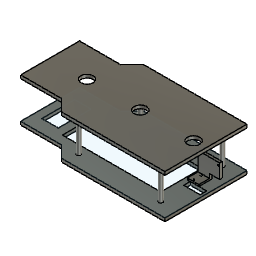
secondbody_final (Autodesk Fusion 360 design; units mm, degrees)
Autodesk Fusion 360 part; units mm, degrees
sketch "Sketch1" plane through (0, 0, 0) normal (0, 0, 1) x (1, 0, 0)
  line L0 (70, 50) -> (-70, 50)
  line L1 (-70, 50) -> (-70, -50)
  line L2 (-70, -50) -> (70, -50)
  line L3 (70, -50) -> (70, 50)
  line L4 (70, 50) -> (-70, -50) construction
  line L5 (-70, 50) -> (70, -50) construction
  line L6 (-70, 35.8825) -> (-120, 35.8825)
  line L7 (-120, 35.8825) -> (-120, -35.8857)
  line L8 (-120, -35.8857) -> (-70, -35.8857)
  line L9 (-70, -35.8857) -> (-70, 35.8825)
  line L10 (-70, 35.8825) -> (-120, -35.8857) construction
  line L11 (-120, 35.8825) -> (-70, -35.8857) construction
  point P0 (-95, -0.0016)
  dimension "d1" = 140
  dimension "d44" = 100
  dimension "d45" = 50
  constraint horizontal L0
  constraint perpendicular L0 L1
  constraint parallel L0 L2
  constraint parallel L1 L3
  constraint coincident L4 origin
  constraint coincident L5 origin
  constraint horizontal L6
  constraint perpendicular L6 L7
  constraint parallel L6 L8
  constraint parallel L7 L9
  constraint coincident L10 P0
  constraint coincident L11 P0
  constraint coincident L1 L6.start
  measures "d1" distance of L1.end L2.end
  measures "d44" distance of L0.start L2.end
  measures "d45" distance of L7.end L8.end
extrude "Extrude1" add sketch "Sketch1" along normal blind 4 makes body 1
sketch "Sketch3" plane through (0, 0, 4) normal (0, 0, 1) x (-1, 0, 0)
  line L0 (70, -50) -> (70, -35.8825)
  line L1 (70, 35.8857) -> (70, 50)
  line L2 (70, 50) -> (-70, 50)
  line L3 (-70, 50) -> (-70, -50)
  line L4 (-70, -50) -> (70, -50)
  line L5 (70, -35.8825) -> (120, -35.8825)
  line L6 (120, -35.8825) -> (120, 35.8857)
  line L7 (120, 35.8857) -> (70, 35.8857)
  line L8 (-40, -25) -> (80, -25)
  line L9 (80, -25) -> (80, 25)
  line L10 (80, 25) -> (-40, 25)
  line L11 (-40, 25) -> (-40, -25)
  line L12 (-40, -25) -> (80, 25) construction
  line L13 (80, -25) -> (-40, 25) construction
  point P0 (20, 0)
  dimension "d54" = 120
  dimension "d55" = 50
  constraint horizontal L8
  constraint perpendicular L8 L9
  constraint parallel L8 L10
  constraint parallel L9 L11
  constraint coincident L12 P0
  constraint coincident L13 P0
  measures "d54" distance of L9.end L10.end
  measures "d55" distance of L8.end L9.end
sketch "Sketch8" plane through (0, 0, 4) normal (0, 0, 1) x (-1, 0, 0)
  line L0 (-70, 50) -> (-70, -50)
  line L1 (-70, -50) -> (70, -50)
  line L2 (70, -50) -> (70, -35.8825)
  line L3 (70, -35.8825) -> (120, -35.8825)
  line L4 (120, -35.8825) -> (120, 35.8857)
  line L5 (120, 35.8857) -> (70, 35.8857)
  line L6 (70, 35.8857) -> (70, 50)
  line L7 (70, 50) -> (-70, 50)
  line L8 (90, 20) -> (90, -20)
  line L9 (90, -20) -> (110, -20)
  line L10 (110, -20) -> (110, 20)
  line L11 (110, 20) -> (90, 20)
  line L12 (90, 20) -> (110, -20) construction
  line L13 (90, -20) -> (110, 20) construction
  point P0 (100, 0)
  dimension "d46" = 40
  dimension "d47" = 20
  constraint perpendicular L8 L9
  constraint parallel L8 L10
  constraint parallel L9 L11
  constraint coincident L12 P0
  constraint coincident L13 P0
  measures "d46" distance of L9.end L10.end
  measures "d47" distance of L8.end L9.end
extrude "Extrude9" cut sketch "Sketch8" against normal blind 45 contours L8 L9 L10 L11 bodies 1
chamfer "Chamfer5" distance 14.1 angle 45 1 edges at (-70, -50, 2) on bodies 1
chamfer "Chamfer6" distance 14.1 angle 45 1 edges at (-70, 50, 2) on bodies 1
sketch "Sketch9" plane through (0, 0, 4) normal (0, 0, 1) x (-1, 0, 0)
  line L0 (55.9, -50) -> (70, -35.9)
  line L1 (70, -35.9) -> (70, -35.8825)
  line L2 (70, -35.8825) -> (120, -35.8825)
  line L3 (120, -35.8825) -> (120, 35.8857)
  line L4 (120, 35.8857) -> (70, 35.8857)
  line L5 (70, 35.8857) -> (70, 35.9)
  line L6 (70, 35.9) -> (55.9, 50)
  line L7 (55.9, 50) -> (-70, 50)
  line L8 (-70, 50) -> (-70, -50)
  line L9 (-70, -50) -> (55.9, -50)
  line L10 (90, -20) -> (90, 20)
  line L11 (90, 20) -> (110, 20)
  line L12 (110, 20) -> (110, -20)
  line L13 (110, -20) -> (90, -20)
extrude "Extrude10" cut sketch "Sketch3" against normal blind 70 contours L8 L9 L10 L11 bodies 1
sketch "Sketch10" plane through (0, 0, 4) normal (0, 0, 1) x (-1, 0, 0)
  line L0 (-44.5, 0) -> (-54.5, 0)
  line L1 (-54.5, 0) -> (-54.5, -20)
  line L2 (-54.5, -20) -> (-44.5, -20)
  line L3 (-44.5, -20) -> (-44.5, 0)
  line L4 (-44.5, 0) -> (-54.5, -20) construction
  line L5 (-54.5, 0) -> (-44.5, -20) construction
  point P0 (-49.5, -10)
  dimension "d58" = 10
  dimension "d59" = 20
  constraint horizontal L0
  constraint perpendicular L0 L1
  constraint parallel L0 L2
  constraint parallel L1 L3
  constraint coincident L4 P0
  constraint coincident L5 P0
  measures "d58" distance of L1.end L2.end
  measures "d59" distance of L0.end L1.end
extrude "Extrude1'" add sketch "Sketch10" along normal blind 2 separate body makes body 2 in component "Component"
sketch "Sketch11" plane through (0, 0, 4) normal (0, 0, 1) x (-1, 0, 0)
  line L0 (-47, 4) -> (-67, 4)
  line L1 (-67, 4) -> (-67, -4)
  line L2 (-67, -4) -> (-47, -4)
  line L3 (-47, -4) -> (-47, 4)
  line L4 (-47, 4) -> (-67, -4) construction
  line L5 (-67, 4) -> (-47, -4) construction
  point P0 (-57, 0)
  dimension "d62" = 20
  dimension "d63" = 8
  constraint horizontal L0
  constraint perpendicular L0 L1
  constraint parallel L0 L2
  constraint parallel L1 L3
  constraint coincident L4 P0
  constraint coincident L5 P0
  measures "d62" distance of L1.end L2.end
  measures "d63" distance of L0.end L1.end
extrude "Extrude11" cut sketch "Sketch11" against normal blind 14 bodies 1
sketch "Sketch12" plane through (0, 0, 6) normal (0, 0, 1) x (-1, 0, 0)
  line L0 (-44.5, -20) -> (-44.5, 0)
  line L1 (-44.5, 0) -> (-54.5, 0)
  line L2 (-54.5, 0) -> (-54.5, -20)
  line L3 (-54.5, -20) -> (-44.5, -20)
  circle A0 centre (-49.5, -6) radius 1
  circle A1 centre (-49.5, -15) radius 1
  dimension "d66" = 2
  dimension "d67" = 2
  measures "d66" diameter of A0
  measures "d67" diameter of A1
extrude "Extrude12" [suppressed]
extrude "Extrude2" cut sketch "Sketch12" against normal blind 2 contours A0 | A1 bodies 2 in component "Component"
sketch "Sketch13" plane through (0, 0, 6) normal (0, 0, 1) x (-1, 0, 0)
  circle A0 centre (-49.5, -15) radius 1
  circle A1 centre (-49.5, -6) radius 1
  line L0 (-44.5, -20) -> (-44.5, 0)
  line L1 (-44.5, 0) -> (-54.5, 0)
  line L2 (-54.5, 0) -> (-54.5, -20)
  line L3 (-54.5, -20) -> (-44.5, -20)
  line L4 (-54.5, -20) -> (-44.5, -20)
  line L5 (-44.5, -20) -> (-44.5, -16.9663)
  line L6 (-44.5, -16.9663) -> (-54.5, -16.9663)
  line L7 (-54.5, -16.9663) -> (-54.5, -20)
  constraint horizontal L4
  constraint vertical L5
  constraint horizontal L6
  constraint vertical L7
  constraint coincident L0 L5.end
  constraint coincident L2.end L3.start
extrude "Extrude3" add sketch "Sketch13" along normal blind 35 contours L0 L2 L3 L4 L5 L6 L7 bodies 2 in component "Component"
sketch "Sketch14" plane through (54.5, 0, 0) normal (1, 0, 0) x (0, 1, 0)
  line L0 (0, 4) -> (20, 4)
  line L1 (20, 4) -> (20, 41)
  line L2 (20, 41) -> (16.9663, 41)
  line L3 (16.9663, 41) -> (16.9663, 6)
  line L4 (16.9663, 6) -> (0, 6)
  line L5 (0, 6) -> (0, 4)
  line L6 (16.9663, 41) -> (20, 41)
  line L7 (20, 41) -> (20, 11)
  line L8 (20, 11) -> (16.9663, 11)
  line L9 (16.9663, 11) -> (16.9663, 41)
  constraint horizontal L6
  constraint vertical L7
  constraint horizontal L8
  constraint vertical L9
  constraint coincident L1 L7.end
  constraint coincident L2.end L3.start
extrude "Extrude4" add sketch "Sketch14" along normal blind 20 contours L1 L2 L3 L6 L7 L8 L9 bodies 2 in component "Component"
sketch "Sketch15" plane through (0, 16.9663, 0) normal (0, -1, 0) x (1, 0, 0)
  line L0 (44.5, 6) -> (54.5, 6)
  line L1 (54.5, 6) -> (54.5, 11)
  line L2 (54.5, 11) -> (74.5, 11)
  line L3 (74.5, 11) -> (74.5, 41)
  line L4 (74.5, 41) -> (44.5, 41)
  line L5 (44.5, 41) -> (44.5, 6)
  circle A0 centre (45, 25) radius 1
  circle A1 centre (68, 25) radius 1
  dimension "d76" = 2
  dimension "d77" = 2
  measures "d76" diameter of A0
  measures "d77" diameter of A1
extrude "Extrude5" add 1 faces at (54.5, 18.9888, 7) along direction (1, 0, 0) blind 3 on bodies 2 bodies 2 in component "Component"
extrude "Extrude6" add 1 faces at (44.5, 18.9888, 17) along direction (-1, 0, 0) blind 3 on bodies 2 bodies 2 in component "Component"
extrude "Extrude7" cut 1 faces at (41.5, 18.9888, 17) along direction (1, 0, 0) blind 2 on bodies 2 bodies 2 in component "Component"
extrude "Extrude8" cut 1 faces at (64.1667, 18.9888, 41) along direction (0, 0, -1) blind 12.5 on bodies 2 bodies 2 in component "Component"
extrude "Extrude9'" cut 1 faces at (74.5, 18.9888, 16.8333) along direction (-1, 0, 0) blind 4.5 on bodies 2 bodies 2 in component "Component"
extrude "Extrude10'" cut 1 faces at (52.8333, 0, 4.6667) along direction (0, 1, 0) blind 4 on bodies 2 bodies 2 in component "Component"
sketch "Sketch16" plane through (0, 0, 4) normal (0, 0, 1) x (-1, 0, 0)
  circle A0 centre (50, -40) radius 2.5
  circle A1 centre (50, 35) radius 2.5
  circle A2 centre (-50, 35) radius 2.5
  circle A3 centre (-50, -40) radius 2.5
  dimension "d90" = 5
  dimension "d91" = 5
  dimension "d92" = 5
  dimension "d93" = 5
  measures "d90" diameter of A0
  measures "d91" diameter of A1
  measures "d92" diameter of A2
  measures "d93" diameter of A3
extrude "Extrude13" add sketch "Sketch16" along normal blind 35 separate body makes body 3 at (51.3564, -32.8999, 27.3333) makes body 4 at (47.5124, 40.2489, 27.3333) makes body 5 at (-48.6436, -32.8999, 27.3333) makes body 6 at (-52.4876, 40.2489, 27.3333)
extrude "Extrude14" add 4 faces at (-50.6608, 39.652, 39) (-50.6608, -35.348, 39) (49.3392, -35.348, 39) (49.3392, 39.652, 39) along direction (0, 0, 1) blind 10 on bodies 3 4 5 6 bodies 3 1 5 6 4
copy_body "CopyPasteBodies1" bodies 1 makes body 7
move_body "Move1" bodies 7 to x (1, 0, 0) y (0, 1, 0) z (0, 0, 1) at (0, 0, 49)
sketch "Sketch17" plane through (0, 0, 53) normal (0, 0, 1) x (-1, 0, 0)
  line L0 (-67, 4) -> (-47, 4)
  line L1 (-47, 4) -> (-47, -4)
  line L2 (-47, -4) -> (-67, -4)
  line L3 (-67, -4) -> (-67, 4)
  line L4 (80, -25) -> (-40, -25)
  line L5 (-40, -25) -> (-40, 25)
  line L6 (-40, 25) -> (80, 25)
  line L7 (80, 25) -> (80, -25)
  line L8 (55.9, -50) -> (70, -35.9)
  line L9 (70, -35.9) -> (70, -35.8825)
  line L10 (70, -35.8825) -> (120, -35.8825)
  line L11 (120, -35.8825) -> (120, 35.8857)
  line L12 (120, 35.8857) -> (70, 35.8857)
  line L13 (70, 35.8857) -> (70, 35.9)
  line L14 (70, 35.9) -> (55.9, 50)
  line L15 (55.9, 50) -> (-70, 50)
  line L16 (-70, 50) -> (-70, -50)
  line L17 (-70, -50) -> (55.9, -50)
  line L18 (90, -20) -> (90, 20)
  line L19 (90, 20) -> (110, 20)
  line L20 (110, 20) -> (110, -20)
  line L21 (110, -20) -> (90, -20)
  line L22 (115, -30) -> (-68.0047, -30)
  line L23 (-68.0047, -30) -> (-68.0047, 29.0941)
  line L24 (-68.0047, 29.0941) -> (115, 29.0941)
  line L25 (115, 29.0941) -> (115, -30)
  constraint horizontal L22
  constraint vertical L23
  constraint horizontal L24
  constraint vertical L25
extrude "Extrude15" add sketch "Sketch17" against normal blind 4 contours L0 L1 L2 L3 | L4 L5 L6 L7 | L18 L19 L20 L21 | L22 L23 L24 L25 bodies 7
sketch "Sketch18" plane through (0, 0, 53) normal (0, 0, 1) x (-1, 0, 0)
  line L0 (55.9, -50) -> (70, -35.9)
  line L1 (70, -35.9) -> (70, -35.8825)
  line L2 (70, -35.8825) -> (120, -35.8825)
  line L3 (120, -35.8825) -> (120, 35.8857)
  line L4 (120, 35.8857) -> (70, 35.8857)
  line L5 (70, 35.8857) -> (70, 35.9)
  line L6 (70, 35.9) -> (55.9, 50)
  line L7 (55.9, 50) -> (-70, 50)
  line L8 (-70, 50) -> (-70, -50)
  line L9 (-70, -50) -> (55.9, -50)
  circle A0 centre (75, 0) radius 7.5
  circle A1 centre (10, 0) radius 7.5
  circle A2 centre (-55, 0) radius 7.5
  dimension "d100" = 15
  dimension "d101" = 15
  dimension "d102" = 15
  measures "d100" diameter of A0
  measures "d101" diameter of A1
  measures "d102" diameter of A2
extrude "Extrude16" cut sketch "Sketch18" against normal blind 5 contours A0 | A1 | A2 bodies 7
extrude "Extrude11'" cut sketch "Sketch15" against normal blind 4 contours L5 A0 | L5 A0 | A1 bodies 2 in component "Component"
component "Component" placed x (1, 0, 0) y (0, 1, 0) z (0, 0, 1) at (0, 0, 0)
